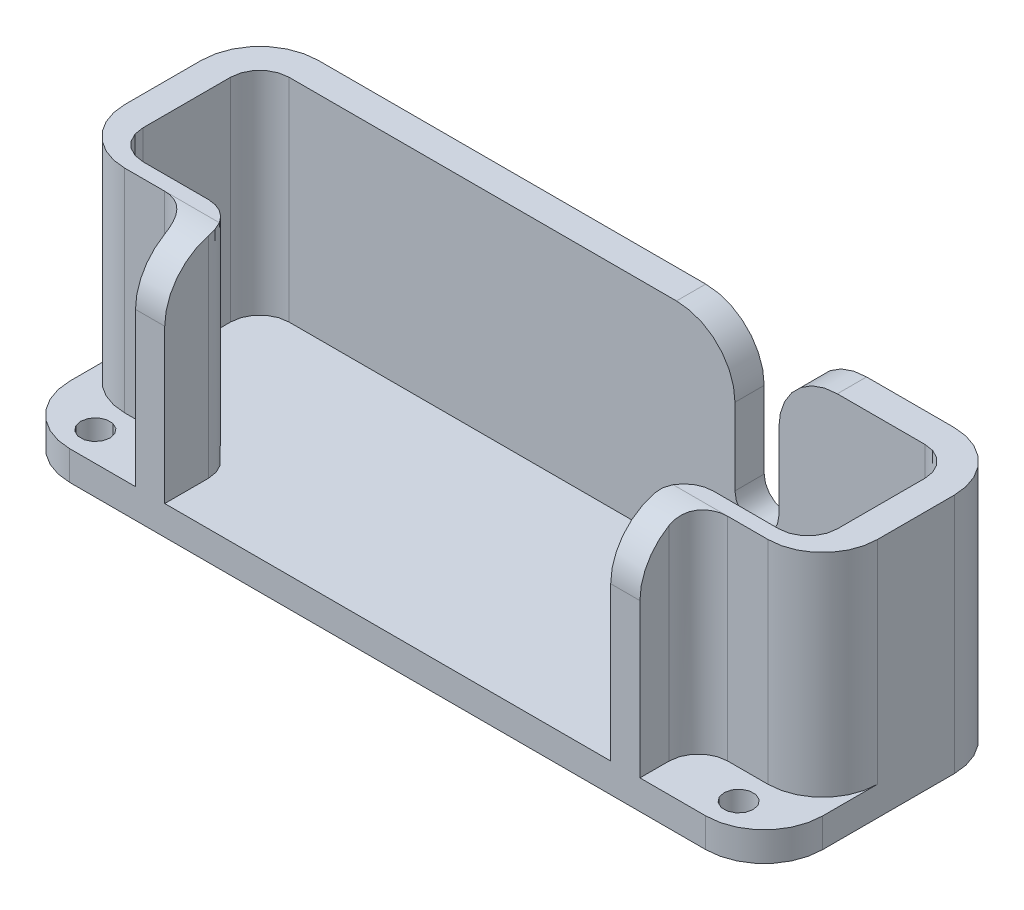
# Autodesk Inventor part: CameraHolder
Saved by Autodesk Inventor 2023 (Build 270158000, 158)
## iProperties
Created: 2022-10-07
Part Number: CameraHolder
Material: Generic
Document SubType Name: Modeling
Designer: deli
Density: 1 g/cm^3
Appearance: Default
Author: deli
Autodesk Inventor part; units mm, degrees
ref_plane "YZ Plane" through (0, 0, 0) normal (1, 0, 0) x (0, 1, 0)
ref_plane "XZ Plane" through (0, 0, 0) normal (0, 1, 0) x (-1, 0, 0)
ref_plane "XY Plane" through (0, 0, 0) normal (0, 0, 1) x (1, 0, 0)
sketch "Sketch1" plane through (0, 0, 0) normal (0, 1, 0) x (-1, 0, 0)
  line L0 (-59.6946, 46.1235) -> (-59.6946, 26.1235)
  line L1 (35.3054, 26.1235) -> (35.3054, 46.1235)
  line L2 (18.3054, 56.1235) -> (18.3054, 46.1235)
  line L3 (18.3054, 46.1235) -> (35.3054, 46.1235)
  line L4 (-42.6946, 56.1235) -> (-42.6946, 46.1235)
  line L5 (-42.6946, 46.1235) -> (-59.6946, 46.1235)
  line L6 (-63.6946, 56.1235) -> (-63.6946, 22.1235)
  line L7 (39.3054, 22.1235) -> (39.3054, 56.1235)
  line L8 (39.3054, 56.1235) -> (18.3054, 56.1235)
  line L9 (-42.6946, 56.1235) -> (-63.6946, 56.1235)
  line L10 (-29.6946, 26.1235) -> (-29.6946, 22.1235)
  line L11 (-35.6946, 26.1235) -> (-35.6946, 22.1235)
  line L12 (-59.6946, 26.1235) -> (-35.6946, 26.1235)
  line L13 (-29.6946, 26.1235) -> (35.3054, 26.1235)
  line L14 (-63.6946, 22.1235) -> (-35.6946, 22.1235)
  line L15 (-29.6946, 22.1235) -> (39.3054, 22.1235)
  point P0 (0, 0)
  dimension "d0" = 95
  dimension "d2" = 17
  dimension "d4" = 17
  dimension "d8" = 4
  dimension "d10" = 4
  dimension "d11" = 10
  dimension "d12" = 10
  dimension "d13" = 6
  dimension "d14" = 28
  dimension "d33" = 20
  dimension "d34" = 0
  dimension "d35" = 4
  dimension "d36" = 4
  dimension "d37" = 20
  constraints: 32 end point, 7 parallel, 4 perpendicular, 2 horizontal
  measures "d0" distance of L1.start L0.end
  measures "d2" distance of L1.end L2.end
  measures "d4" distance of L0.start L4.end
  measures "d8" distance between parallel lines of L1 L7
  measures "d10" distance between parallel lines of L0 L6
  measures "d11" distance between parallel lines of L5 L9
  measures "d12" distance between parallel lines of L3 L8
  measures "d13" distance between parallel lines of L11 L10
  measures "d14" distance between parallel lines of L11 L6
  measures "d33" distance of L1.start L1.end
  measures "d34" distance between parallel lines of L14 L15
  measures "d35" distance between parallel lines of L15 L13
  measures "d36" distance between parallel lines of L14 L12
  measures "d37" distance between parallel lines of L12 L5
extrude "Extrusion1" add sketch "Sketch1" along normal blind 29
sketch "Sketch2" plane through (0, 0, 0) normal (0, -1, 0) x (1, 0, 0)
  line L0 (-39.3054, 56.1235) -> (-18.3054, 56.1235) projected
  line L1 (63.6946, 22.1235) -> (35.6946, 22.1235) projected
  line L2 (-39.3054, 56.1235) -> (63.6946, 56.1235)
  line L3 (63.6946, 56.1235) -> (63.6946, 22.1235)
  line L4 (63.6946, 22.1235) -> (-39.3054, 22.1235)
  line L5 (-39.3054, 22.1235) -> (-39.3054, 56.1235)
  point P0 (0, 0)
  point P1 (-18.3054, 56.1235)
  constraints: 8 end point, 2 parallel, 1 horizontal, 1 perpendicular
extrude "Extrusion2" add sketch "Sketch2" along normal blind 4
sketch "Sketch3" plane through (0, 0, 0) normal (0, 1, 0) x (1, 0, 0)
  line L0 (29.6946, -26.1235) -> (29.6946, -22.1235) projected
  line L1 (35.6946, -22.1235) -> (35.6946, -26.1235) projected
  line L2 (29.6946, -26.1235) -> (35.6946, -26.1235)
  line L3 (35.6946, -26.1235) -> (35.6946, -22.1235)
  line L4 (35.6946, -22.1235) -> (29.6946, -22.1235)
  line L5 (29.6946, -22.1235) -> (29.6946, -26.1235)
  point P0 (0, 0)
  point P1 (35.6946, -26.1235)
  point P2 (29.6946, -22.1235)
  constraints: 8 end point, 2 parallel, 1 horizontal, 1 perpendicular
extrude "Extrusion3" add sketch "Sketch3" along normal blind 7.5
fillet "Fillet1" radius 3 2 edges at (29.6946, 7.5, 24.1235) (35.6946, 7.5, 24.1235)
fillet "Fillet2" radius 4 6 edges at (-35.3054, 14.5, 26.1235) (-35.3054, 14.5, 46.1235) (59.6946, 14.5, 26.1235) (59.6946, 14.5, 46.1235) (-18.3054, 14.5, 46.1235) (42.6946, 14.5, 46.1235)
sketch "Sketch4" plane through (0, 29, 0) normal (0, 1, 0) x (1, 0, 0)
  circle A0 centre (-31.8054, -52.1235) radius 2
  circle A1 centre (56.1946, -52.1235) radius 2
  line L0 (-39.3054, -56.1235) -> (-18.3054, -56.1235) projected
  line L1 (-22.3054, -46.1235) -> (-31.3054, -46.1235) projected
  line L2 (42.6946, -56.1235) -> (63.6946, -56.1235) projected
  line L3 (-39.3054, -22.1235) -> (-39.3054, -56.1235) projected
  line L4 (63.6946, -56.1235) -> (63.6946, -22.1235) projected
  point P0 (0, 0)
  point P1 (-18.3054, -46.1235)
  dimension "d23" = 4
  dimension "d24" = 4
  dimension "d25" = 10
  dimension "d26" = 4
  dimension "d27" = 4
  dimension "d28" = 88
  dimension "d29" = 7.5
  dimension "d30" = 103
  constraints: 2 centre point
  measures "d23" diameter of A0
  measures "d24" diameter of A1
  measures "d25" distance between parallel lines of L0 L1
  measures "d26" distance from line of A0.centre L0
  measures "d27" distance from line of L2 A1.centre
  measures "d28" distance of A1.centre A0.centre
  measures "d29" distance from line of A0.centre L3
  measures "d30" distance between parallel lines of L4 L3
extrude "Extrusion4" cut sketch "Sketch4" against normal blind 40
sketch "Sketch5" plane through (0, 29, 0) normal (0, 1, 0) x (1, 0, 0)
  circle A0 centre (-31.8054, -52.1235) radius 2 projected
  circle A1 centre (-31.8054, -52.1235) radius 4
  circle A2 centre (56.1946, -52.1235) radius 2 projected
  circle A3 centre (56.1946, -52.1235) radius 4
  arc A4 (-39.3054, -40.6235) -> (-31.8054, -48.1235) centre (-31.8054, -40.6235) ccw
  line L0 (-39.3054, -22.1235) -> (-39.3054, -56.1235) projected
  line L1 (-39.3054, -56.1235) -> (-18.3054, -56.1235) projected
  line L2 (-18.3054, -56.1235) -> (-18.3054, -50.1235) projected
  arc A5 (-22.3054, -52.1235) -> (-26.3054, -48.1235) centre (-26.3054, -52.1235) ccw
  line L3 (-31.8054, -48.1235) -> (-26.3054, -48.1235)
  line L4 (-22.3054, -52.1235) -> (-22.3054, -56.1235)
  line L5 (63.6946, -56.1235) -> (-39.3054, -56.1235) projected
  circle A6 centre (56.1946, -40.6235) radius 7.5
  arc A7 (50.6946, -48.1235) -> (46.6946, -52.1235) centre (50.6946, -52.1235) ccw
  line L6 (46.6946, -52.1235) -> (46.6946, -56.1235)
  line L7 (50.6946, -48.1235) -> (56.1946, -48.1235)
  line L8 (63.6946, -56.1235) -> (63.6946, -22.1235) projected
  line L9 (42.6946, -50.1235) -> (42.6946, -56.1235) projected
  point P0 (0, 0)
  point P1 (63.6946, -40.6235)
  point P2 (56.1946, -48.1235)
  dimension "d38" = 8
  dimension "d39" = 8
  dimension "d40" = 8
  dimension "d44" = 4
  dimension "d45" = 4
  dimension "d46" = 4
  dimension "d47" = 8
  dimension "d48" = 4
  dimension "d49" = 4
  dimension "d50" = 4
  constraints: 8 end point, 6 point on circle, 6 tangent, 4 centre point, 2 coincident, 2 vertical alignment, 1 horizontal, 1 perpendicular, 1 point on line, 1 vertical, 9 other
  measures "d40" distance edge to line of A4 L1
  measures "d44" radius of A5
  measures "d45" distance edge to line of A5 L2
  measures "d48" radius of A7
  measures "d50" distance between parallel lines of L6 L9
extrude "Extrusion5" cut sketch "Sketch5" against normal blind 29 contours A0 | A1 | A1 L3 A5 L4 L1 | A1 L1 L0 A4 | A2 | A3 | A3 A6 L8 L5 | A3 L5 L6 A7 L7
fillet "Fillet3" radius 8 8 edges at (-39.3054, -2, 56.1235) (63.6946, -2, 56.1235) (63.6946, 12.5, 22.1235) (-39.3054, 12.5, 22.1235) (29.6946, 29, 24.1235) (35.6946, 29, 24.1235) (44.6946, 29, 56.1235) (-20.3054, 29, 56.1235)
equation "\"d4\" = d2"
equation "\"d10\" = d8"
equation "\"d12\" = d11"
equation "\"d36\" = d35"
equation "\"d37\" = d33"
equation "\"d24\" = d23"
equation "\"d27\" = d26"
equation "\"d29\" = -0.5 * d28 + 0.5 * d30"
equation "\"d39\" = d38"
equation "\"d40\" = d38"
equation "\"d44\" = 0.5 * d38"
equation "\"d46\" = d44"
equation "\"d47\" = d39"
equation "\"d48\" = 0.5 * d39"
equation "\"d49\" = d48"
equation "\"d50\" = d49"
equation "\"d9\" = d8"
equation "\"d43\" = d40"
body "Solid1"
